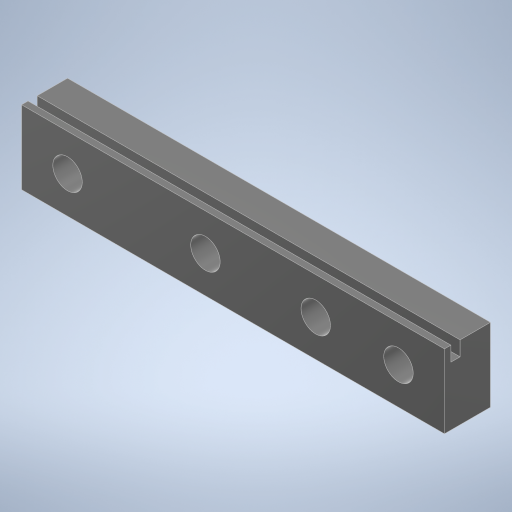
# Autodesk Inventor part: cutter_stopper
Saved by Autodesk Inventor 2024 (Build 280153000, 153)
## iProperties
Created: 2025-06-02
Part Number: cutter_stopper
Material: ABS プラスチック
Document SubType Name: Modeling
Designer: 1412z
Density: 1.06 g/cm^3
Appearance: 滑らか - 黒
Author: 1412z
Autodesk Inventor part; units mm, degrees
ref_plane "YZ Plane" through (0, 0, 0) normal (1, 0, 0) x (0, 1, 0)
ref_plane "XZ Plane" through (0, 0, 0) normal (0, 1, 0) x (-1, 0, 0)
ref_plane "XY Plane" through (0, 0, 0) normal (0, 0, 1) x (1, 0, 0)
sketch "スケッチ1" plane through (0, 0, 0) normal (0, 0, 1) x (1, 0, 0)
  line L0 (10, -2) -> (-10, -2)
  line L1 (-10, -2) -> (-10, 2)
  line L2 (-10, 2) -> (10, 2)
  line L3 (10, 2) -> (10, -2)
  line L4 (10, -2) -> (-10, 2) construction
  line L5 (-10, -2) -> (10, 2) construction
  point P0 (0, 0)
  dimension "d0" = 20
  dimension "d1" = 4
  constraints: 12 end point, 2 midpoint, 2 parallel, 1 horizontal, 1 perpendicular
  measures "d0" distance of L1.end L2.end
  measures "d1" distance of L0.end L1.end
extrude "押し出し1" add sketch "スケッチ1" along normal blind 2.5
sketch "スケッチ2" plane through (-10, 2, 0) normal (0, 1, 0) x (1, 0, 0)
  line L0 (0, -1.9) -> (20, -1.9)
  line L1 (20, 0) -> (20, -2.5) projected
  line L2 (20, -1.9) -> (20, -1.65)
  line L3 (20, -1.65) -> (0, -1.65)
  line L4 (0, -1.65) -> (0, -2.15)
  line L5 (0, -2.15) -> (20, -2.15)
  line L6 (20, -2.15) -> (20, -1.9)
  point P0 (10, 0)
  dimension "d4" = 0.25
  dimension "d5" = 0.5
  dimension "d12" = 20
  dimension "d13" = 20
  constraints: 12 end point, 3 point on line, 2 perpendicular, 1 collinear, 1 horizontal, 1 parallel
  measures "d4" distance of L0.end L2.end
  measures "d5" distance of L3.end L4.end
  measures "d12" distance of L2.end L3.end
  measures "d13" distance of L0.start L0.end
extrude "押し出し2" cut sketch "スケッチ2" against normal blind 0.5
sketch "スケッチ3" plane through (0, 0, 0) normal (0, 0, -1) x (-1, 0, 0)
  circle A0 centre (3, 0) radius 0.8
  circle A1 centre (-3, 0) radius 0.8
  point P0 (0, 0)
  dimension "d8" = 1.6
  dimension "d9" = 1.6
  constraints: 2 centre point
  measures "d8" diameter of A0
  measures "d9" diameter of A1
extrude "押し出し3" cut sketch "スケッチ3" against normal blind 5
sketch "スケッチ5" plane through (-10, -2, 0) normal (-1, 0, 0) x (0, 0, 1)
  line L0 (0, 0) -> (2.5, 0) projected
  line L1 (0, 4) -> (1.65, 4) projected
  line L2 (0, 0) -> (0, 4)
  line L3 (1.65, 3.5) -> (1.65, 4) projected
  line L4 (0, 4) -> (1.65, 4)
  line L5 (1.65, 4) -> (1.65, 3.5)
  line L6 (2.15, 4) -> (2.15, 3.5) projected
  line L7 (1.65, 3.5) -> (2.15, 3.5)
  line L8 (2.15, 3.5) -> (2.15, 4)
  line L9 (2.5, 0) -> (2.5, 4) projected
  line L10 (2.15, 4) -> (2.5, 4)
  line L11 (2.5, 4) -> (2.5, 0)
  line L12 (2.5, 0) -> (0, 0)
  point P0 (0, 2)
  constraints: 16 end point, 5 perpendicular, 3 collinear
extrude "押し出し5" add sketch "スケッチ5" along normal blind 3
sketch "スケッチ6" plane through (0, 0, 2.5) normal (0, 0, 1) x (1, 0, 0)
  circle A0 centre (7.5, 0) radius 0.8
  circle A1 centre (-10.5, 0) radius 0.8
  point P0 (0, 0)
  dimension "d20" = 1.6
  dimension "d21" = 1.6
  constraints: 2 centre point
  measures "d20" diameter of A0
  measures "d21" diameter of A1
extrude "押し出し6" cut sketch "スケッチ6" against normal blind 3
sketch "スケッチ7" plane through (10, -2, 0) normal (1, 0, 0) x (0, 0, -1)
  line L0 (-2.15, 3.5) -> (-2.15, 4) projected
  line L1 (-2.15, 4) -> (-2.15, 3.2)
  line L2 (-2.15, 3.2) -> (-1.65, 3.2)
  line L3 (-1.65, 4) -> (-1.65, 3.5) projected
  line L4 (-1.65, 3.2) -> (-1.65, 4)
  line L5 (-1.65, 4) -> (-2.15, 4)
  point P0 (0, 2)
  dimension "d24" = 0.8
  constraints: 8 end point, 2 collinear, 2 perpendicular
  measures "d24" distance of L0.end L1.end
extrude "押し出し7" cut sketch "スケッチ7" against normal blind 30
